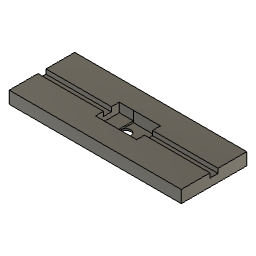
simple_extruder_holder v4 (Autodesk Fusion 360 design; units mm, degrees)
Autodesk Fusion 360 part; units mm, degrees
sketch "Sketch1" plane through (0, 0, 0) normal (0, 0, 1) x (1, 0, 0)
  line L0 (-85.8321, 26.0818) -> (124.3679, 26.0818)
  line L1 (124.3679, 26.0818) -> (124.3679, -53.9182)
  line L2 (124.3679, -53.9182) -> (-85.8321, -53.9182)
  line L3 (-85.8321, -53.9182) -> (-85.8321, 26.0818)
  dimension "d1" = 210.2
  dimension "d2" = 80
  constraint horizontal L0
  constraint vertical L1
  constraint horizontal L2
  constraint vertical L3
  measures "d1" distance of L0.start L0.end
  measures "d2" distance of L0.start L2.end
extrude "Extrude1" add sketch "Sketch1" along normal blind 40
sketch "Sketch2" plane through (0, 0, 40) normal (0, 0, 1) x (-1, 0, 0)
  line L0 (85.8321, 53.9182) -> (-124.3679, 53.9182)
  line L1 (-124.3679, 53.9182) -> (-124.3679, -26.0818)
  line L2 (-124.3679, -26.0818) -> (85.8321, -26.0818)
  line L3 (85.8321, -26.0818) -> (85.8321, 53.9182)
  line L4 (85.8321, -26.0818) -> (-124.3679, -26.0818)
  line L5 (-124.3679, -26.0818) -> (-124.3679, -17.0818)
  line L6 (-124.3679, -17.0818) -> (85.8321, -17.0818)
  line L7 (85.8321, -17.0818) -> (85.8321, -26.0818)
  dimension "d5" = 210.2
  dimension "d6" = 9
  constraint horizontal L4
  constraint vertical L5
  constraint horizontal L6
  constraint vertical L7
  constraint coincident L2.end L3.start
  measures "d5" distance of L2.end L1.end
  measures "d6" distance of L2.end L6.end
move_body "Move1" bodies 1 to x (1, 0, 0) y (0, 1, 0) z (0, 0, 1) at (0, 35.5, 0)
extrude "Extrude2" cut sketch "Sketch2" against normal blind 5 contours L1 L2 L3 L4 L5 L6 L7
sketch "Sketch3" plane through (0, 0, 40) normal (0, 0, 1) x (-1, 0, 0)
  line L0 (85.8321, -26.0818) -> (-124.3679, -26.0818)
  line L1 (-124.3679, -26.0818) -> (-124.3679, -61.5818)
  line L2 (-124.3679, -61.5818) -> (85.8321, -61.5818)
  line L3 (85.8321, -61.5818) -> (85.8321, -26.0818)
sketch "Sketch4" plane through (0, 0, 40) normal (0, 0, 1) x (-1, 0, 0)
move_body "Move2" bodies 1 to x (1, 0, 0) y (0, 1, 0) z (0, 0, 1) at (0, -35.5, 0)
sketch "Sketch5" plane through (0, 0, 0) normal (0, 0, 1) x (1, 0, 0)
  line L0 (44.3679, -28.4182) -> (-5.8321, -28.4182)
  line L1 (-5.8321, -28.4182) -> (-5.8321, 0.5818)
  line L2 (-5.8321, 0.5818) -> (44.3679, 0.5818)
  line L3 (44.3679, 0.5818) -> (44.3679, -28.4182)
  dimension "d9" = 50.2
  dimension "d10" = 29
  constraint horizontal L0
  constraint vertical L1
  constraint horizontal L2
  constraint vertical L3
  measures "d9" distance of L0.start L0.end
  measures "d10" distance of L0.start L2.end
move_body "Move3" bodies 1 to x (1, 0, 0) y (0, 1, 0) z (0, 0, 1) at (0, 0, -40)
extrude "Extrude3" cut sketch "Sketch5" against normal blind 6.15
sketch "Sketch6" plane through (0, 0, 0) normal (0, 0, 1) x (1, 0, 0)
  line L0 (44.3717, -28.4047) -> (11.3717, -28.4047)
  line L1 (11.3717, -28.4047) -> (11.3717, 0.5953)
  line L2 (11.3717, 0.5953) -> (44.3717, 0.5953)
  line L3 (44.3717, 0.5953) -> (44.3717, -28.4047)
  dimension "d13" = 33
  dimension "d14" = 29
  constraint horizontal L0
  constraint vertical L1
  constraint horizontal L2
  constraint vertical L3
  measures "d13" distance of L0.start L0.end
  measures "d14" distance of L0.start L2.end
extrude "Extrude4" cut sketch "Sketch6" against normal blind 8.1
extrude "Extrude5" add 1 faces at (97.7025, 5.753, 0) along direction (0, 0, 1) blind 5
extrude "Extrude6" add 1 faces at (-59.1655, -33.5848, 0) along direction (0, 0, 1) blind 5
extrude "Extrude7" add 1 faces at (71.0371, -15.4182, -5) along direction (0, 0, 1) blind 5
extrude "Extrude8" add 1 faces at (-59.1655, -12.4182, -5) along direction (0, 0, 1) blind 5
sketch "Sketch7" plane through (0, 0, 5) normal (0, 0, 1) x (-1, 0, 0)
  line L0 (-44.3717, -0.5953) -> (-44.3717, 9.4182)
  line L1 (-44.3717, 9.4182) -> (-124.3679, 9.4182)
  line L2 (-124.3679, 9.4182) -> (-124.3679, -26.0818)
  line L3 (-124.3679, -26.0818) -> (85.8321, -26.0818)
  line L4 (85.8321, -26.0818) -> (85.8321, 9.4182)
  line L5 (85.8321, 9.4182) -> (5.8321, 9.4182)
  line L6 (5.8321, 9.4182) -> (5.8321, -0.5818)
  line L7 (5.8321, -0.5818) -> (-11.3717, -0.5818)
  line L8 (-11.3717, -0.5818) -> (-11.3717, -0.5953)
  line L9 (-11.3717, -0.5953) -> (-44.3717, -0.5953)
sketch "Sketch8" plane through (0, 0, 5) normal (0, 0, 1) x (-1, 0, 0)
  line L0 (-44.3717, -0.5953) -> (-44.3717, 9.4182)
  line L1 (-44.3717, 9.4182) -> (-124.3679, 9.4182)
  line L2 (-124.3679, 9.4182) -> (-124.3679, -26.0818)
  line L3 (-124.3679, -26.0818) -> (85.8321, -26.0818)
  line L4 (85.8321, -26.0818) -> (85.8321, 4.4182)
  line L5 (85.8321, 9.4182) -> (5.8321, 9.4182)
  line L6 (5.8321, 9.4182) -> (5.8321, -0.5818)
  line L7 (5.8321, -0.5818) -> (-11.3717, -0.5818)
  line L8 (-11.3717, -0.5818) -> (-11.3717, -0.5953)
  line L9 (-11.3717, -0.5953) -> (-44.3717, -0.5953)
  line L10 (85.8321, 9.4182) -> (-124.8914, 9.4182)
  line L11 (-124.8914, 9.4182) -> (-124.8914, 19.4182)
  line L12 (-124.8914, 19.4182) -> (85.8321, 19.4182)
  line L13 (85.8321, 19.4182) -> (85.8321, 9.4182)
  dimension "d25" = 10
  constraint horizontal L10
  constraint vertical L11
  constraint horizontal L12
  constraint vertical L13
  constraint coincident L5.start L10.start
  measures "d25" distance of L5.start L12.end
move_body "Move4" bodies 1 to x (1, 0, 0) y (0, 1, 0) z (0, 0, 1) at (0, 0.5, 0)
move_body "Move5" bodies 1 to x (1, 0, 0) y (0, 1, 0) z (0, 0, 1) at (0, -1, 0)
extrude "Extrude9" cut sketch "Sketch8" against normal blind 5.5 contours L1 L5 L10 L11 L12 L13
extrude "Extrude10" cut 1 faces at (-15.7655, -1.0848, -40) along direction (0, 0, 1) blind 30
sketch "Sketch9" plane through (0, 0, 5) normal (0, 0, 1) x (-1, 0, 0)
  line L0 (85.8321, 9.4182) -> (5.8321, 9.4182)
  line L1 (5.8321, 9.4182) -> (5.8321, -0.0818)
  line L2 (5.8321, -0.0818) -> (-11.3717, -0.0818)
  line L3 (-11.3717, -0.0818) -> (-11.3717, -0.0953)
  line L4 (-11.3717, -0.0953) -> (-44.3717, -0.0953)
  line L5 (-44.3717, -0.0953) -> (-44.3717, 9.4182)
  line L6 (-44.3717, 9.4182) -> (-124.3679, 9.4182)
  line L7 (-124.3679, 9.4182) -> (-124.3679, -25.5818)
  line L8 (-124.3679, -25.5818) -> (85.8321, -25.5818)
  line L9 (85.8321, -25.5818) -> (85.8321, 9.4182)
  circle A0 centre (-17.4118, 15.0021) radius 6
  dimension "d30" = 12
  measures "d30" diameter of A0
extrude "Extrude11" cut sketch "Sketch9" against normal blind 58 contours A0
extrude "Extrude12" add 1 faces at (-32.4988, -19.4182, 1.3333) along direction (0, 1, 0) blind 0.1
extrude "Extrude13" add 1 faces at (97.7025, -19.4182, 3.1667) along direction (0, 1, 0) blind 0.1
extrude "Extrude14" add 1 faces at (71.0371, -9.4182, 3.1667) along direction (0, -1, 0) blind 0.1
extrude "Extrude15" add 1 faces at (-59.1655, -9.4182, 3.1667) along direction (0, -1, 0) blind 0.1
